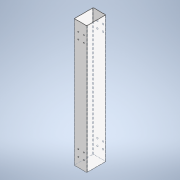
# Autodesk Inventor part: tubo3-40x80x800
Saved by Autodesk Inventor 2021 (Build 250183000, 183)
## iProperties
Created: 2026-05-19
Part Number: tubo3-40x80x800
Material: Acero, carbono
Document SubType Name: Modeling
Designer: nelso
Density: 7.85 g/cm^3
Appearance: Blanco
Author: nelso
Autodesk Inventor part; units mm, degrees
ref_plane "YZ Plane" through (0, 0, 0) normal (1, 0, 0) x (0, 1, 0)
ref_plane "XZ Plane" through (0, 0, 0) normal (0, 1, 0) x (-1, 0, 0)
ref_plane "XY Plane" through (0, 0, 0) normal (0, 0, 1) x (1, 0, 0)
sketch "Sketch2" plane through (0, 0, 0) normal (0, 1, 0) x (-1, 0, 0)
  line L0 (-40, 60) -> (40, 60)
  line L1 (40, 60) -> (40, -60)
  line L2 (40, -60) -> (-40, -60)
  line L3 (-40, -60) -> (-40, 60)
  line L4 (-40, 60) -> (40, -60) construction
  line L5 (40, 60) -> (-40, -60) construction
  line L6 (-37.76, 57.76) -> (37.76, 57.76)
  line L7 (37.76, 57.76) -> (37.76, -57.76)
  line L8 (37.76, -57.76) -> (-37.76, -57.76)
  line L9 (-37.76, -57.76) -> (-37.76, 57.76)
  line L10 (-37.76, 57.76) -> (37.76, -57.76) construction
  line L11 (37.76, 57.76) -> (-37.76, -57.76) construction
  point P0 (0, 0)
  dimension "d8" = 80
  dimension "d9" = 120
  dimension "d10" = 75.52
  dimension "d61" = 115.52
  constraints: 24 end point, 4 midpoint, 4 parallel, 2 horizontal, 2 perpendicular
  measures "d8" distance of L1.end L2.end
  measures "d9" distance of L0.end L1.end
  measures "d10" distance of L7.end L8.end
  measures "d61" distance of L6.end L7.end
extrude "Extrusion2" add sketch "Sketch2" along normal mid plane 790
fillet "Fillet2" radius 4 4 edges at (-40, 0, 60) (40, 0, 60) (40, 0, -60) (-40, 0, -60)
fillet "Fillet2" radius 2 4 edges at (37.76, 0, 57.76) (-37.76, 0, -57.76) (37.76, 0, -57.76) (-37.76, 0, 57.76)
sketch "Sketch13" plane through (-36, 395, 60) normal (0, 0, 1) x (1, 0, 0)
  circle A0 centre (44.0231, -99.3) radius 3.35 projected
  circle A1 centre (9.0231, -99.3) radius 3.35 projected
  circle A2 centre (9.0231, -57.9) radius 3.35 projected
  circle A3 centre (44.0231, -57.9) radius 3.35 projected
  circle A4 centre (44.0231, -690.7) radius 3.35 projected
  circle A5 centre (44.0231, -732.1) radius 3.35 projected
  circle A6 centre (9.0231, -732.1) radius 3.35 projected
  circle A7 centre (9.0231, -690.7) radius 3.35 projected
  point P0 (36, -395)
extrude "Extrusion13" cut sketch "Sketch13" against normal through all
sketch "Sketch14" plane through (36, 395, -60) normal (0, 0, -1) x (-1, 0, 0)
  circle A0 centre (27.9769, -732.1) radius 3.35 projected
  circle A1 centre (27.9769, -732.1) radius 5
  circle A2 centre (27.9769, -690.7) radius 3.35 projected
  circle A3 centre (27.9769, -690.7) radius 5
  circle A4 centre (62.9769, -690.7) radius 3.35 projected
  circle A5 centre (62.9769, -690.7) radius 5
  circle A6 centre (48.9769, -732.1) radius 5
  circle A7 centre (27.9769, -57.9) radius 3.35 projected
  circle A8 centre (27.9769, -57.9) radius 5
  circle A9 centre (62.9769, -99.3) radius 3.35 projected
  circle A10 centre (62.9769, -99.3) radius 5
  circle A11 centre (62.9769, -57.9) radius 3.35 projected
  circle A12 centre (62.9769, -57.9) radius 5
  circle A13 centre (27.9769, -99.3) radius 3.35 projected
  circle A14 centre (27.9769, -99.3) radius 5
  point P0 (36, -395)
  point P1 (0, -693.8899)
  point P2 (0, -687.5101)
  dimension "d64" = 10
  dimension "d65" = 10
  dimension "d66" = 10
  dimension "d67" = 10
  dimension "d68" = 10
  dimension "d69" = 10
  dimension "d70" = 10
  dimension "d71" = 10
  constraints: 8 centre point, 7 coincident, 1 other
  measures "d64" diameter of A1
  measures "d65" diameter of A3
  measures "d66" diameter of A5
  measures "d67" diameter of A6
  measures "d68" diameter of A8
  measures "d69" diameter of A10
  measures "d70" diameter of A12
  measures "d71" diameter of A14
extrude "Extrusion14" cut sketch "Sketch14" against normal blind 10 contours A1 | A3 | A4 | A5 | A6 | A8 | A10 | A12 | A14
body "Solid2"
